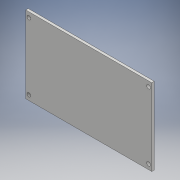
# Autodesk Inventor part: FSCase_Battery_Cover_v6
Saved by Autodesk Inventor 2017 (Build 210142000, 142)
## iProperties
Created: 2020-03-12
Part Number: FSCase_Battery_Cover_v6
Material: Generic
Document SubType Name: Modeling
Designer: Manny
Density: 1 g/cm^3
Appearance: Default
Author: Manny
Autodesk Inventor part; units mm, degrees
ref_plane "YZ Plane" through (0, 0, 0) normal (1, 0, 0) x (0, 1, 0)
ref_plane "XZ Plane" through (0, 0, 0) normal (0, 1, 0) x (-1, 0, 0)
ref_plane "XY Plane" through (0, 0, 0) normal (0, 0, 1) x (1, 0, 0)
sketch "Sketch1" plane through (0, 0, 0) normal (0, 1, 0) x (-1, 0, 0)
  line L0 (0, -61) -> (-100, -61)
  line L1 (-100, -61) -> (-100, 0)
  line L2 (-100, 0) -> (0, 0)
  line L3 (0, 0) -> (0, -61)
  dimension "d0" = 100
  dimension "d1" = 61
  constraints: 8 end point, 2 parallel, 1 horizontal, 1 perpendicular
  measures "d0" distance of L1.end L2.end
  measures "d1" distance of L0.end L1.end
extrude "Extrusion1" add sketch "Sketch1" along normal blind 2
sketch "Sketch2" plane through (0, 2, 0) normal (0, 1, 0) x (1, 0, 0)
  circle A0 centre (97.5, 57) radius 1.5
  circle A1 centre (97.5, 4) radius 1.5
  circle A2 centre (2.5, 4) radius 1.5
  circle A3 centre (2.5, 57) radius 1.5
  line L0 (100, 0) -> (100, 61) projected
  line L1 (100, 61) -> (0, 61) projected
  line L2 (0, 0) -> (100, 0) projected
  line L3 (0, 61) -> (0, 0) projected
  dimension "d4" = 2.5
  dimension "d5" = 4
  dimension "d6" = 3
  dimension "d7" = 2.5
  dimension "d8" = 4
  dimension "d9" = 4
  dimension "d10" = 2.5
  dimension "d11" = 4
  dimension "d12" = 2.5
  constraints: 4 centre point, 3 equal radius
  measures "d4" distance from line of L0 A0.centre
  measures "d5" distance from line of L1 A0.centre
  measures "d6" diameter of A0
  measures "d7" distance from line of L0 A1.centre
  measures "d8" distance from line of L2 A1.centre
  measures "d9" distance from line of L2 A2.centre
  measures "d10" distance from line of L3 A2.centre
  measures "d11" distance from line of L1 A3.centre
  measures "d12" distance from line of L3 A3.centre
extrude "Extrusion2" cut sketch "Sketch2" against normal blind 4 contours A0 | A1 | A2 | A3
body "Solid1"
